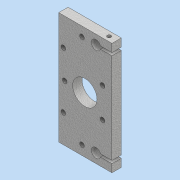
# Autodesk Inventor part: Podstawa górna osi Z
Saved by Autodesk Inventor 2018 (Build 220112000, 112)
## iProperties
Created: 2019-02-01
Part Number: Podstawa górna osi Z
Material: Ogólny
Document SubType Name: Modeling
Designer: Dawid
Density: 1 g/cm^3
Appearance: Aluminium odlewane
Author: Dawid
Autodesk Inventor part; units mm, degrees
ref_plane "YZ Plane" through (0, 0, 0) normal (1, 0, 0) x (0, 1, 0)
ref_plane "XZ Plane" through (0, 0, 0) normal (0, 1, 0) x (-1, 0, 0)
ref_plane "XY Plane" through (0, 0, 0) normal (0, 0, 1) x (1, 0, 0)
sketch "Szkic10" plane through (0, 0, 0) normal (0, 1, 0) x (-1, 0, 0)
  line L0 (-25, 60) -> (25, 60)
  line L1 (25, 60) -> (25, -60)
  line L2 (25, -60) -> (-25, -60)
  line L3 (-25, -60) -> (-25, 60)
  line L4 (-25, 60) -> (25, -60) construction
  line L5 (25, 60) -> (-25, -60) construction
  point P0 (0, 0)
  dimension "d75" = 50
  dimension "d76" = 120
  constraints: 12 end point, 2 midpoint, 2 parallel, 1 horizontal, 1 perpendicular
  measures "d75" distance of L1.end L2.end
  measures "d76" distance of L0.end L1.end
extrude "Wyciągnięcie proste6" add sketch "Szkic10" along normal blind 10
sketch "Szkic11" plane through (-25, 0, -60) normal (-1, 0, 0) x (0, 0, 1)
  line L0 (120, 0) -> (0, 0) projected
  line L1 (120, 0) -> (120, 10) projected
  line L2 (0, 10) -> (120, 10) projected
  line L3 (0, 0) -> (0, 10) projected
  line L4 (0, 0) -> (120, 0) projected
  line L5 (0, 0) -> (0, 5)
  line L6 (0, 5) -> (120, 5)
  line L7 (0, 5) -> (20, 5)
  line L8 (20, 5) -> (40, 5)
  line L9 (40, 5) -> (80, 5)
  line L10 (80, 5) -> (100, 5)
  circle A0 centre (20, 5) radius 2.5
  circle A1 centre (40, 5) radius 2.5
  circle A2 centre (80, 5) radius 2.5
  circle A3 centre (100, 5) radius 2.5
  point P0 (60, 0)
  dimension "d79" = 5
  dimension "d80" = 20
  dimension "d81" = 20
  dimension "d84" = 5
  dimension "d85" = 5
  dimension "d86" = 5
  dimension "d87" = 5
  dimension "d105" = 20
  dimension "d106" = 20
  constraints: 12 end point, 4 centre point, 4 coincident, 4 point on line, 2 midpoint
  measures "d79" distance of L0.end L5.end
  measures "d80" distance of L5.end L7.end
  measures "d81" distance of L7.end L8.end
  measures "d84" diameter of A0
  measures "d85" diameter of A1
  measures "d86" diameter of A2
  measures "d87" diameter of A3
  measures "d105" distance from line of L1 L10.end
  measures "d106" distance of L10.end A2.centre
extrude "Wyciągnięcie proste7" cut sketch "Szkic11" against normal blind 20 contours A3 L6 | L6 A3 | A0 L6 | L6 A0 | A2 L6 | L6 A2 | A1 L6 | L6 A1
sketch "Szkic12" plane through (0, 10, 0) normal (0, 1, 0) x (1, 0, 0)
  line L0 (25, -60) -> (25, 60) projected
  line L1 (25, 0) -> (3, 0)
  circle A0 centre (3, 0) radius 13
  point P0 (0, 0)
  dimension "d102" = 22
  dimension "d103" = 26
  constraints: 2 end point, 1 centre point, 1 coincident, 1 horizontal, 1 midpoint
  measures "d102" distance of L1.start L1.end
  measures "d103" diameter of A0
extrude "Wyciągnięcie proste8" cut sketch "Szkic12" against normal up to next
sketch "Szkic13" plane through (0, 0, 0) normal (0, -1, 0) x (1, 0, 0)
  line L0 (25, 60) -> (-25, 60) projected
  line L1 (-25, 60) -> (-25, -60) projected
  line L2 (-25, -60) -> (25, -60) projected
  line L3 (25, -60) -> (25, 60) projected
  line L4 (25, 60) -> (25, 50)
  line L5 (25, -60) -> (25, 60) projected
  line L6 (25, 50) -> (-25, 50)
  line L7 (25, -60) -> (25, -50)
  line L8 (25, -50) -> (-25, -50)
  line L9 (25, 50) -> (15, 50)
  line L10 (25, -50) -> (15, -50)
  circle A0 centre (15, 50) radius 5
  circle A1 centre (15, -50) radius 5
  point P0 (0, 0)
  dimension "d93" = 10
  dimension "d94" = 10
  dimension "d95" = 10
  dimension "d96" = 10
  dimension "d97" = 10
  dimension "d98" = 10
  constraints: 12 end point, 6 point on line, 2 centre point, 2 coincident, 2 perpendicular
  measures "d93" distance of L0.start L4.end
  measures "d94" distance of L2.end L7.end
  measures "d95" distance of L4.end L9.end
  measures "d96" distance of L7.end L10.end
  measures "d97" diameter of A0
  measures "d98" diameter of A1
extrude "Wyciągnięcie proste9" cut sketch "Szkic13" against normal blind 3 contours A0 L6 | L6 A0 | A1 L8 | L8 A1
sketch "Szkic14" plane through (15, 3, -50) normal (0, -1, 0) x (1, 0, 0)
  circle A0 centre (0, 0) radius 5 projected
  circle A1 centre (0, 100) radius 5 projected
  point P0 (-15, 50)
extrude "Wyciągnięcie proste10" cut sketch "Szkic14" against normal blind 10
sketch "Szkic15" plane through (25, 0, 60) normal (1, 0, 0) x (0, 0, -1)
  line L0 (120, 0) -> (0, 0) projected
  line L1 (120, 0) -> (120, 10) projected
  line L2 (0, 10) -> (120, 10) projected
  line L3 (0, 0) -> (0, 10) projected
  point P0 (60, 0)
extrude "Wyciągnięcie proste11" add sketch "Szkic15" along normal blind 7
sketch "Szkic16" plane through (-25, 0, 60) normal (0, 0, 1) x (1, 0, 0)
  line L0 (57, 0) -> (0, 0) projected
  line L1 (57, 10) -> (57, 0) projected
  line L2 (0, 10) -> (57, 10) projected
  line L3 (0, 0) -> (0, 10) projected
  line L4 (35, 10) -> (45, 10) projected
  line L5 (45, 0) -> (35, 0) projected
  line L6 (53, 0) -> (45, 0)
  line L7 (57, 0) -> (0, 0) projected
  line L8 (45, 0) -> (45, 10)
  line L9 (0, 10) -> (57, 10) projected
  line L10 (57, 10) -> (57, 0) projected
  line L11 (53, 5) -> (45, 5)
  line L12 (45, 5) -> (49, 5)
  circle A0 centre (49, 5) radius 2
  line L13 (49, 5) -> (53, 5)
  line L14 (53, 5) -> (53, 10)
  line L15 (53, 5) -> (53, 0)
  point P0 (25, 0)
  dimension "d113" = 4
  dimension "d114" = 4
  dimension "d115" = 5
  dimension "d116" = 45
  dimension "d117" = 4
  constraints: 14 end point, 3 perpendicular, 2 midpoint, 2 point on line, 1 centre point, 1 coincident, 1 collinear
  measures "d113" distance of L11.end L12.end
  measures "d114" diameter of A0
  measures "d115" distance between parallel lines of L2 L11
  measures "d116" distance between parallel lines of L3 L8
  measures "d117" distance of L11.start L13.start
sketch "Szkic17" plane through (-25, 0, -60) normal (0, 0, -1) x (-1, 0, 0)
  line L0 (-53, 10) -> (0, 10)
  line L1 (-53, 0) -> (-53, 10)
  line L2 (0, 0) -> (-53, 0)
  line L3 (0, 10) -> (0, 0)
  line L4 (-35, 0) -> (-45, 0)
  line L5 (-45, 10) -> (-35, 10)
  line L6 (-53, 10) -> (-45, 10)
  line L7 (-53, 10) -> (0, 10)
  line L8 (-45, 10) -> (-45, 0)
  line L9 (0, 0) -> (-53, 0)
  line L10 (-53, 0) -> (-53, 10)
  line L11 (-53, 5) -> (-45, 5)
  line L12 (-45, 5) -> (-49, 5)
  circle A0 centre (-49, 5) radius 2
  line L13 (-49, 5) -> (-53, 5)
  line L14 (-53, 5) -> (-53, 0)
  line L15 (-53, 5) -> (-53, 10)
  line L16 (0, 0) -> (-57, 0) projected
  line L17 (0, 0) -> (0, 10) projected
  point P0 (-25, 0)
  point P1 (-25, 10)
  dimension "d119" = 4
  dimension "d120" = 4
  dimension "d121" = 5
  dimension "d122" = 45
  dimension "d123" = 4
  constraints: 32 end point, 3 perpendicular, 2 midpoint, 2 point on line, 1 centre point, 1 coincident, 1 collinear
  measures "d119" distance of L11.end L12.end
  measures "d120" diameter of A0
  measures "d121" distance between parallel lines of L2 L11
  measures "d122" distance between parallel lines of L3 L8
  measures "d123" distance of L11.start L13.start
hole "Otwór4" at (24, 5, -60) direction (0, 0, 1) diameter 4 depth 20 tip angle 118
hole "Otwór5" at (24, 5, 60) direction (0, 0, -1) diameter 4 depth 20 tip angle 118
sketch "Szkic18" plane through (0, 0, 0) normal (0, -1, 0) x (1, 0, 0)
  circle A0 centre (15, -50) radius 5 projected
  circle A1 centre (15, 50) radius 5 projected
  circle A2 centre (3, 0) radius 13 projected
  line L0 (32, 60) -> (-25, 60) projected
  line L1 (-25, 60) -> (-25, -60) projected
  line L2 (-25, -60) -> (32, -60) projected
  line L3 (32, 60) -> (32, -60) projected
  line L4 (15, -50) -> (32, -50)
  line L5 (15, 50) -> (32, 50)
  line L6 (32, -60) -> (32, 60) projected
  line L7 (15, 50) -> (15, 51.5)
  line L8 (15, 51.5) -> (32, 51.5)
  line L9 (15, 50) -> (15, 48.5)
  line L10 (15, 48.5) -> (32, 48.5)
  line L11 (15, -50) -> (15, -48.5)
  line L12 (15, -48.5) -> (32, -48.5)
  line L13 (15, -50) -> (15, -51.5)
  line L14 (15, -51.5) -> (32, -51.5)
  point P0 (0, 0)
  dimension "d138" = 1.5
  dimension "d139" = 1.5
  dimension "d140" = 1.5
  dimension "d141" = 1.5
  constraints: 20 end point, 9 point on line, 4 perpendicular, 1 horizontal, 1 parallel, 1 vertical
  measures "d138" distance of L5.start L7.end
  measures "d139" distance of L5.start L9.end
  measures "d140" distance of L4.start L11.end
  measures "d141" distance of L4.start L13.end
extrude "Wyciągnięcie proste12" cut sketch "Szkic18" against normal up to next contours L4 L11 L12 A0 | L4 L3 L14 A0 | A0 L14 L13 L4 | A0 L12 L3 L4 | L10 A1 L5 L3 | L5 A1 L8 L3 | L10 L9 L5 A1 | L5 L7 L8 A1
thread "Gwint9" size "M5x0.8" class "6H" standard "ANSI Metric M Profile" full length
thread "Gwint10" size "M5x0.8" class "6H" standard "ANSI Metric M Profile" full length
thread "Gwint11" size "M5x0.8" class "6H" standard "ANSI Metric M Profile" full length
thread "Gwint12" size "M5x0.8" class "6H" standard "ANSI Metric M Profile" full length
sketch "Szkic20" plane through (0, 0, 0) normal (0, -1, 0) x (1, 0, 0)
  line L0 (32, 48.5) -> (32, -48.5) projected
  line L1 (-25, 60) -> (-25, -60) projected
  circle A0 centre (3, 0) radius 13 projected
  circle A1 centre (22, 16) radius 2.5
  circle A2 centre (22, -16) radius 2.5
  circle A3 centre (-18.5, 0) radius 2.5
  circle A4 centre (3, 0) radius 15
  line L2 (-25, 25) -> (-25, -25)
  line L3 (-25, -25) -> (32, -25)
  line L4 (32, -25) -> (32, 25)
  line L5 (32, 25) -> (-25, 25)
  point P0 (0, 0)
  constraints: 8 end point, 4 centre point
extrude "Wyciągnięcie proste14" cut sketch "Szkic20" against normal up to next contours A1 | A2 | A3
thread "Gwint13" size "M5x0.8" class "6H" standard "ANSI Metric M Profile" full length
thread "Gwint14" size "M5x0.8" class "6H" standard "ANSI Metric M Profile" full length
thread "Gwint15" size "M5x0.8" class "6H" standard "ANSI Metric M Profile" full length
sketch "Szkic21" plane through (0, 10, 0) normal (0, 1, 0) x (1, 0, 0)
  line L0 (32, 48.5) -> (32, -48.5)
  line L1 (32, -51.5) -> (32, -60)
  line L2 (32, 60) -> (32, 30)
  line L3 (-25, -60) -> (-25, 60)
  line L4 (-25, -60) -> (32, -60)
  line L5 (-25, 60) -> (32, 60)
  circle A0 centre (0, 50) radius 2.5
  circle A1 centre (-20, 30) radius 2.5
  circle A2 centre (-20, -30) radius 2.5
  circle A3 centre (0, -50) radius 2.5
  line L6 (-25, -60) -> (32, -60) projected
  line L7 (32, -51.5) -> (32, -60) projected
  point P0 (0, 0)
  constraints: 12 end point, 4 centre point
extrude "Wyciągnięcie proste15" cut sketch "Szkic21" against normal up to next
thread "Gwint16" size "M5x0.8" class "6H" standard "ANSI Metric M Profile" full length
thread "Gwint17" size "M5x0.8" class "6H" standard "ANSI Metric M Profile" full length
thread "Gwint18" size "M5x0.8" class "6H" standard "ANSI Metric M Profile" full length
thread "Gwint19" size "M5x0.8" class "6H" standard "ANSI Metric M Profile" full length
